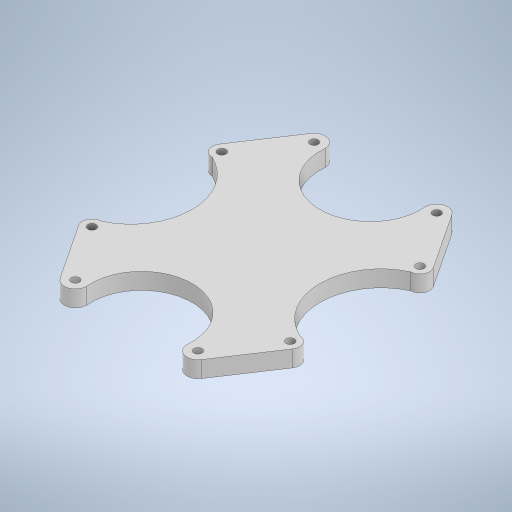
# Autodesk Inventor part: Part1
Saved by Autodesk Inventor 2023 (Build 270158000, 158)
## iProperties
Created: 2023-01-25
Part Number: Part1
Material: Generic
Document SubType Name: Modeling
Designer: Steven
Density: 1 g/cm^3
Appearance: Default
Author: Steven
Autodesk Inventor part; units mm, degrees
ref_plane "YZ Plane" through (0, 0, 0) normal (1, 0, 0) x (0, 1, 0)
ref_plane "XY Plane" through (0, 0, 0) normal (0, 0, 1) x (1, 0, 0)
sketch "Sketch1" plane through (0, 0, 0) normal (0, 1, 0) x (-1, 0, 0)
  arc A0 (29.0364, 11.5992) -> (31.5928, 13.9152) centre (6.8441, 38.6639) ccw
  line L0 (31.5928, 13.9152) -> (38.8388, 21.1612)
  arc A1 (38.8388, 21.1612) -> (31.6005, 42.3971) centre (30, 30) ccw
  spline S0 degree 2 poles (31.6005, 42.3971) (29.6875, 43.0872) (28.5558, 43.5262) knots 0 0 0 1 1 1 weights 1 1.23412 1.413428
  arc A2 (26.4074, 45.5015) -> (28.5558, 43.5262) centre (30.0023, 47.2554) ccw
  arc A3 (26.4074, 45.5015) -> (17.8643, 43.6369) centre (22.363, 43.5284) ccw
  spline S1 degree 2 poles (17.8643, 43.6369) (16.884, 36.226) (10.7077, 28.418) knots 0 0 0 1.796523 1.796523 1.796523 weights 1 2.961796 1.074949
  arc A4 (8.2725, 26.0348) -> (10.7077, 28.418) centre (3.309, 33.5424) ccw
  arc A5 (-8.2725, 26.0348) -> (8.2725, 26.0348) centre (0, 38.5475) ccw
  arc A6 (-10.7077, 28.418) -> (-8.2725, 26.0348) centre (-3.309, 33.5424) ccw
  spline S2 degree 2 poles (-10.7077, 28.418) (-16.884, 36.226) (-17.8643, 43.6369) knots -1.796523 -1.796523 -1.796523 0 0 0 weights 1.074949 2.961796 1
  arc A7 (-17.8643, 43.6369) -> (-26.4074, 45.5015) centre (-22.363, 43.5284) ccw
  arc A8 (-28.5558, 43.5262) -> (-26.4074, 45.5015) centre (-30.0023, 47.2554) ccw
  spline S3 degree 2 poles (-28.5558, 43.5262) (-29.6875, 43.0872) (-31.6005, 42.3971) knots 0 0 0 1 1 1 weights 1.413428 1.23412 1
  arc A9 (-31.6005, 42.3971) -> (-38.8388, 21.1612) centre (-30, 30) ccw
  line L1 (-38.8388, 21.1612) -> (-31.5928, 13.9152)
  arc A10 (-31.5928, 13.9152) -> (-29.0364, 11.5992) centre (-6.8441, 38.6639) ccw
  arc A11 (-29.0364, -11.5992) -> (-29.0364, 11.5992) centre (-38.5475, 0) ccw
  arc A12 (-29.0364, -11.5992) -> (-31.5928, -13.9152) centre (-6.8441, -38.6639) ccw
  line L2 (-31.5928, -13.9152) -> (-38.8388, -21.1612)
  arc A13 (-38.8388, -21.1612) -> (-31.6005, -42.3971) centre (-30, -30) ccw
  spline S4 degree 2 poles (-31.6005, -42.3971) (-29.6875, -43.0872) (-28.5558, -43.5262) knots 0 0 0 1 1 1 weights 1 1.23412 1.413428
  arc A14 (-26.4074, -45.5015) -> (-28.5558, -43.5262) centre (-30.0023, -47.2554) ccw
  arc A15 (-26.4074, -45.5015) -> (-17.8643, -43.6369) centre (-22.363, -43.5284) ccw
  spline S5 degree 2 poles (-17.8643, -43.6369) (-16.884, -36.226) (-10.7077, -28.418) knots 0 0 0 1.796523 1.796523 1.796523 weights 1 2.961796 1.074949
  arc A16 (-8.2725, -26.0348) -> (-10.7077, -28.418) centre (-3.309, -33.5424) ccw
  arc A17 (8.2725, -26.0348) -> (-8.2725, -26.0348) centre (0, -38.5475) ccw
  arc A18 (10.7077, -28.418) -> (8.2725, -26.0348) centre (3.309, -33.5424) ccw
  spline S6 degree 2 poles (10.7077, -28.418) (16.884, -36.226) (17.8643, -43.6369) knots -1.796523 -1.796523 -1.796523 0 0 0 weights 1.074949 2.961796 1
  arc A19 (17.8643, -43.6369) -> (26.4074, -45.5015) centre (22.363, -43.5284) ccw
  arc A20 (28.5558, -43.5262) -> (26.4074, -45.5015) centre (30.0023, -47.2554) ccw
  spline S7 degree 2 poles (28.5558, -43.5262) (29.6875, -43.0872) (31.6005, -42.3971) knots 0 0 0 1 1 1 weights 1.413428 1.23412 1
  arc A21 (31.6005, -42.3971) -> (38.8388, -21.1612) centre (30, -30) ccw
  line L3 (38.8388, -21.1612) -> (31.5928, -13.9152)
  arc A22 (31.5928, -13.9152) -> (29.0364, -11.5992) centre (6.8441, -38.6639) ccw
  arc A23 (29.0364, 11.5992) -> (29.0364, -11.5992) centre (38.5475, 0) ccw
  circle A24 centre (-36.1224, 23.6779) radius 1.53
  circle A25 centre (36.1224, -23.6779) radius 1.53
  circle A26 centre (-36.1224, -23.6779) radius 1.53
  circle A27 centre (36.1224, 23.6779) radius 1.53
  circle A28 centre (-22.363, -43.5284) radius 1.5
  circle A29 centre (22.363, 43.5284) radius 1.5
  circle A30 centre (22.363, -43.5284) radius 1.5
  circle A31 centre (12.75, -12.75) radius 1.5
  circle A32 centre (-10, -10) radius 1.5
  circle A33 centre (-10, 10) radius 1.5
  circle A34 centre (10, -10) radius 1.5
  circle A35 centre (-12.75, -12.75) radius 1.5
  circle A36 centre (-12.75, 12.75) radius 1.5
  circle A37 centre (12.75, 12.75) radius 1.5
  circle A38 centre (10, 10) radius 1.5
  circle A39 centre (-22.363, 43.5284) radius 1.5
  arc A40 (6.6461, 25.1002) -> (25.1002, 6.6461) centre (12.75, 12.75) ccw construction
  arc A41 (25.1002, -6.6461) -> (6.6461, -25.1002) centre (12.75, -12.75) ccw construction
  arc A42 (-6.6461, -25.1002) -> (-25.1002, -6.6461) centre (-12.75, -12.75) ccw construction
  arc A43 (-25.1002, 6.6461) -> (-6.6461, 25.1002) centre (-12.75, 12.75) ccw construction
  line L4 (0, 0) -> (27.295, 0) construction
  line L5 (0, 0) -> (0, -38.5475) construction
  point P0 (0, 0)
  point P1 (28.5558, 23.5475)
  point P2 (28.5558, -23.5475)
  point P3 (-28.5558, 23.5475)
  point P4 (-28.5558, -23.5475)
  constraints: 64 point on circle, 44 centre point, 12 end point, 4 coincident, 4 tangent, 3 symmetric about line, 1 horizontal, 1 vertical, 146 other
ref_plane "Work Plane1" through (0, 55, 0) normal (0, 1, 0) x (-1, 0, 0)
sketch "Sketch6" plane through (0, 0, 0) normal (0, 1, 0) x (-1, 0, 0)
  circle A0 centre (22.363, 43.5284) radius 1.5 projected
  circle A1 centre (36.1224, 23.6779) radius 1.53 projected
  circle A2 centre (36.1224, -23.6779) radius 1.53 projected
  circle A3 centre (22.363, -43.5284) radius 1.5 projected
  circle A4 centre (-22.363, -43.5284) radius 1.5 projected
  circle A5 centre (-36.1224, 23.6779) radius 1.53 projected
  circle A6 centre (-36.1224, -23.6779) radius 1.53 projected
  circle A7 centre (-22.363, 43.5284) radius 1.5 projected
  circle A8 centre (22.363, 43.5284) radius 4
  circle A9 centre (-22.363, 43.5284) radius 4
  circle A10 centre (-22.363, -43.5284) radius 4
  circle A11 centre (22.363, -43.5284) radius 4
  arc A12 (18.363, -43.5284) -> (-18.363, -43.5284) centre (0, -41.7486) ccw
  line L0 (0, 0) -> (27.295, 0) construction
  circle A13 centre (22.363, 43.5284) radius 1.5
  circle A14 centre (-22.363, 43.5284) radius 1.5
  circle A15 centre (-22.363, 43.5284) radius 4
  circle A16 centre (22.363, 43.5284) radius 4
  arc A17 (-18.363, 43.5284) -> (18.363, 43.5284) centre (0, 41.7486) ccw
  circle A18 centre (36.1224, 23.6779) radius 3.5
  circle A19 centre (36.1224, -23.6779) radius 3.5
  circle A20 centre (-36.1224, -23.6779) radius 3.5
  circle A21 centre (-36.1224, 23.6779) radius 3.5
  arc A22 (36.1224, 20.1779) -> (36.1224, -20.1779) centre (45.6412, 0) ccw
  line L1 (0, 0) -> (0, -38.5475) construction
  arc A23 (-36.1224, -20.1779) -> (-36.1224, 20.1779) centre (-45.6412, 0) ccw
  line L2 (39.0396, -25.6118) -> (25.697, -45.7386)
  line L3 (-39.0396, -25.6118) -> (-25.697, -45.7386)
  line L4 (39.0396, 25.6118) -> (25.697, 45.7386)
  line L5 (-39.0396, 25.6118) -> (-25.697, 45.7386)
  point P0 (0, 0)
  point P1 (30, -30)
  point P2 (-36.1224, 20.1779)
  point P3 (18.363, 43.5284)
  point P4 (-18.363, 43.5284)
  dimension "d12" = 8
  dimension "d14" = 7
  dimension "d10" = 8
  dimension "d11" = 8
  dimension "d13" = 8
  dimension "d15" = 7
  dimension "d16" = 7
  dimension "d17" = 7
  constraints: 16 symmetric about line, 12 centre point, 12 point on circle, 10 coincident, 8 end point, 2 horizontal alignment, 2 tangent, 1 horizontal, 17 other
  measures "d10" diameter of A8
  measures "d11" diameter of A9
  measures "d13" diameter of A11
  measures "d15" diameter of A19
  measures "d16" diameter of A20
  measures "d17" diameter of A21
extrude "Extrusion1" add sketch "Sketch6" along normal blind 6 contours A8 A17 | A8 L4 A18 A22 A19 L2 A11 A12 A10 L3 A20 A23 A21 L5 A9 A17 | A18 | A9 A17 | A19 | A21 | A11 A12 | A20 | A10 A12 picked at (25.4742, 43.0807) picked at (-19.3312, 42.6827) picked at (25.4742, -43.0807) picked at (-19.3312, -42.6827)
body "Solid2"
